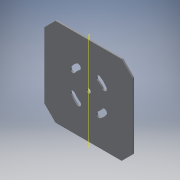
# Autodesk Inventor part: bottom plate
Saved by Autodesk Inventor 2017 (Build 210142000, 142)
## iProperties
Created: 2018-12-02
Part Number: bottom plate
Material: Generic
Document SubType Name: Modeling
Designer: Eric the Great
Density: 1 g/cm^3
Appearance: Default
Author: Eric the Great
Autodesk Inventor part; units mm, degrees
ref_plane "YZ Plane" through (0, 0, 0) normal (1, 0, 0) x (0, 1, 0)
ref_plane "XZ Plane" through (0, 0, 0) normal (0, 1, 0) x (-1, 0, 0)
ref_plane "XY Plane" through (0, 0, 0) normal (0, 0, 1) x (1, 0, 0)
sketch "Sketch1" plane through (0, 0, 0) normal (0, 1, 0) x (-1, 0, 0)
  line L0 (-152.4, 152.4) -> (152.4, 152.4)
  line L1 (152.4, 152.4) -> (152.4, -152.4)
  line L2 (152.4, -152.4) -> (-152.4, -152.4)
  line L3 (-152.4, -152.4) -> (-152.4, 152.4)
  line L4 (-152.4, 152.4) -> (152.4, -152.4) construction
  line L5 (152.4, 152.4) -> (-152.4, -152.4) construction
  line L6 (0, -35) -> (-30.3109, -17.5)
  line L7 (-30.3109, -17.5) -> (-30.3109, 17.5)
  line L8 (-30.3109, 17.5) -> (0, 35)
  line L9 (0, 35) -> (30.3109, 17.5)
  line L10 (30.3109, 17.5) -> (30.3109, -17.5)
  line L11 (30.3109, -17.5) -> (0, -35)
  arc A0 (54.3646, 35.4255) -> (35.7748, 54.1354) centre (0, 0) ccw construction
  arc A1 (61.905, 40.339) -> (40.7367, 61.6439) centre (0, 0) ccw
  arc A2 (46.8242, 30.5119) -> (30.8128, 46.6268) centre (0, 0) ccw
  arc A3 (46.8242, 30.5119) -> (61.905, 40.339) centre (54.3646, 35.4255) ccw
  arc A4 (40.7367, 61.6439) -> (30.8128, 46.6268) centre (35.7748, 54.1354) ccw
  arc A5 (-61.6439, 40.7367) -> (-46.6268, 30.8128) centre (-54.1354, 35.7748) ccw
  arc A6 (-30.5119, 46.8242) -> (-46.6268, 30.8128) centre (0, 0) ccw
  arc A7 (-40.339, 61.905) -> (-61.6439, 40.7367) centre (0, 0) ccw
  arc A8 (-30.5119, 46.8242) -> (-40.339, 61.905) centre (-35.4255, 54.3646) ccw
  arc A9 (-40.7367, -61.6439) -> (-30.8128, -46.6268) centre (-35.7748, -54.1354) ccw
  arc A10 (-46.8242, -30.5119) -> (-30.8128, -46.6268) centre (0, 0) ccw
  arc A11 (-61.905, -40.339) -> (-40.7367, -61.6439) centre (0, 0) ccw
  arc A12 (-46.8242, -30.5119) -> (-61.905, -40.339) centre (-54.3646, -35.4255) ccw
  arc A13 (61.6439, -40.7367) -> (46.6268, -30.8128) centre (54.1354, -35.7748) ccw
  arc A14 (30.5119, -46.8242) -> (46.6268, -30.8128) centre (0, 0) ccw
  arc A15 (40.339, -61.905) -> (61.6439, -40.7367) centre (0, 0) ccw
  arc A16 (30.5119, -46.8242) -> (40.339, -61.905) centre (35.4255, -54.3646) ccw
  circle A17 centre (0, 0) radius 7.5
  dimension "d1" = 304.8
  dimension "d2" = 304.8
  dimension "d5" = 35
  dimension "d11" = 360
  dimension "d13" = 18
  dimension "d14" = 15
  constraints: 34 point on circle, 24 end point, 18 centre point, 4 coincident, 4 tangent, 2 midpoint, 2 parallel, 1 horizontal, 1 perpendicular, 58 other
  measures "d1" distance of L1.end L2.end
  measures "d2" distance of L0.end L1.end
  measures "d5" distance of L9.end L10.end
  measures "d13" radial gap between concentric circles of A1 A2
  measures "d14" diameter of A17
extrude "Extrusion1" add sketch "Sketch1" along normal blind 5 contours L0 L1 L2 L3 | L6 L7 L8 L9 L10 L11
chamfer "Chamfer1" distance 38.1 angle 45 4 edges at (152.4, 2.5, -152.4) (-152.4, 2.5, -152.4) (-152.4, 2.5, 152.4) (152.4, 2.5, 152.4)
ref_plane "Work Plane1" through (0, 0, -17.5) normal (1, 0, 0) x (0, 0, -1)
body "Solid1"
